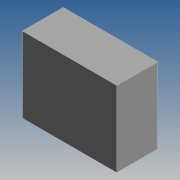
# Autodesk Inventor part: R005
Saved by Autodesk Inventor 2017 (Build 210142000, 142)
## iProperties
Created: 2018-10-05
Part Number: R005
Material: Acier / Stahl
Document SubType Name: Modeling
Designer: Gilles Mottiez
Density: 7.85 g/cm^3
Appearance: Par défaut
Description: Port HDMI Raspberry pi 3B
Author: Gilles Mottiez
Autodesk Inventor part; units mm, degrees
ref_plane "YZ Plane" through (0, 0, 0) normal (1, 0, 0) x (0, 1, 0)
ref_plane "XZ Plane" through (0, 0, 0) normal (0, 1, 0) x (-1, 0, 0)
ref_plane "XY Plane" through (0, 0, 0) normal (0, 0, 1) x (1, 0, 0)
sketch "Sketch1" plane through (0, 0, 0) normal (0, 0, 1) x (1, 0, 0)
  line L0 (0, 0) -> (15, 0)
  line L1 (15, 0) -> (15, 6.5)
  line L2 (15, 6.5) -> (0, 6.5)
  line L3 (0, 6.5) -> (0, 0)
  dimension "d0" = 15
  dimension "d1" = 6.5
  constraints: 8 end point, 2 parallel, 1 horizontal, 1 perpendicular
  measures "d0" distance of L2.end L1.end
  measures "d1" distance of L1.end L0.end
extrude "Extrusion1" add sketch "Sketch1" along normal blind 12
